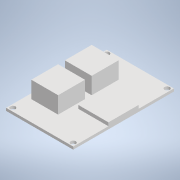
# Autodesk Inventor part: plate
Saved by Autodesk Inventor 2021.2 (Build 252289000, 289)
## iProperties
Created: 2021-11-19
Part Number: plate
Material: Типовые
Document SubType Name: Modeling
Designer: kanad
Density: 1 g/cm^3
Appearance: По умолчанию
Author: kanad
Autodesk Inventor part; units mm, degrees
ref_plane "YZ Plane" through (0, 0, 0) normal (1, 0, 0) x (0, 1, 0)
ref_plane "XZ Plane" through (0, 0, 0) normal (0, 1, 0) x (-1, 0, 0)
ref_plane "XY Plane" through (0, 0, 0) normal (0, 0, 1) x (1, 0, 0)
sketch "Эскиз1" plane through (0, 0, 0) normal (0, 1, 0) x (-1, 0, 0)
  line L0 (0, 0) -> (40, 0)
  line L1 (40, 0) -> (40, -60)
  line L2 (40, -60) -> (0, -60)
  line L3 (0, -60) -> (0, 0)
  line L4 (37, -12) -> (21, -12)
  line L5 (21, -12) -> (21, -28)
  line L6 (21, -28) -> (37, -28)
  line L7 (37, -28) -> (37, -12)
  line L8 (37, -32) -> (21, -32)
  line L9 (21, -32) -> (21, -48)
  line L10 (21, -48) -> (37, -48)
  line L11 (37, -48) -> (37, -32)
  line L12 (0, -21) -> (18, -21)
  line L13 (18, -21) -> (18, -39)
  line L14 (18, -39) -> (0, -39)
  line L15 (0, -39) -> (0, -21)
  circle A0 centre (2, -2) radius 1.5
  circle A1 centre (2, -58) radius 1.5
  circle A2 centre (38, -2) radius 1.5
  circle A3 centre (38, -58) radius 1.5
  point P0 (0, -39)
  dimension "d0" = 40
  dimension "d1" = 60
  dimension "d2" = 16
  dimension "d3" = 16
  dimension "d4" = 3
  dimension "d5" = 12
  dimension "d6" = 16
  dimension "d7" = 16
  dimension "d8" = 4
  dimension "d9" = 3
  dimension "d10" = 18
  dimension "d11" = 18
  dimension "d12" = 21
  dimension "d13" = 3
  dimension "d14" = 2
  dimension "d15" = 2
  dimension "d18" = 56
  dimension "d21" = 36
  constraints: 32 end point, 8 parallel, 5 horizontal, 4 centre point, 4 perpendicular, 1 point on line, 1 vertical, 6 other
  measures "d0" distance of L1.end L2.end
  measures "d1" distance of L0.end L1.end
  measures "d2" distance of L6.end L5.end
  measures "d3" distance of L5.end L4.end
  measures "d4" distance between parallel lines of L1 L7
  measures "d5" distance between parallel lines of L0 L4
  measures "d6" distance of L10.end L9.end
  measures "d7" distance of L9.end L8.end
  measures "d8" distance between parallel lines of L6 L8
  measures "d9" distance between parallel lines of L1 L11
  measures "d10" distance of L13.end L14.end
  measures "d11" distance of L12.end L13.end
  measures "d12" distance between parallel lines of L0 L12
  measures "d13" diameter of A0
  measures "d14" distance from line of L3 A0.centre
  measures "d15" distance from line of L0 A0.centre
  measures "d18" distance of A0.centre A1.centre
  measures "d21" distance of A0.centre A2.centre
extrude "Выдавливание1" add sketch "Эскиз1" along normal blind 1.6 contours L0 L1 L2 L3 L14 L13 L12
extrude "Выдавливание2" add sketch "Эскиз1" along normal blind 11.6 contours L7 L6 L5 L4 | L11 L10 L9 L8
extrude "Выдавливание3" add sketch "Эскиз1" along normal blind 3.6 contours L12 L13 L14 L3
